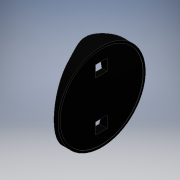
# Autodesk Inventor part: ET15
Saved by Autodesk Inventor 2016 (Build 200138000, 138)
## iProperties
Created: 2016-03-28
Part Number: ET15
Material: Genérico
Document SubType Name: Modeling
Designer: Usuario1
Density: 1 g/cm^3
Appearance: Valor por defecto
Author: Usuario1
Autodesk Inventor part; units mm, degrees
ref_plane "YZ Plane" through (0, 0, 0) normal (1, 0, 0) x (0, 1, 0)
ref_plane "XZ Plane" through (0, 0, 0) normal (0, 1, 0) x (-1, 0, 0)
ref_plane "XY Plane" through (0, 0, 0) normal (0, 0, 1) x (1, 0, 0)
sketch "Boceto4" plane through (0, 0, 0) normal (1, 0, 0) x (0, 1, 0)
  circle A0 centre (0, 0) radius 1.15
  circle A1 centre (0, 0) radius 1.0926
  constraints: 2 centre point
extrude "Extrusión3" add sketch "Boceto4" along normal blind 0.27 and the other way blind 0.155 contours A0 | A1
sketch "Boceto5" plane through (0, 0, 0) normal (0, 1, 0) x (-1, 0, 0)
  line L0 (-0.27, 1.15) -> (-0.27, -1.15) projected
  line L1 (0.155, -1.15) -> (0.155, 1.15) projected
  line L2 (0.155, -1.15) -> (0.155, 1.15) projected
  line L3 (0.155, -1.15) -> (-0.27, -1.15) projected
  line L4 (0.155, 1.15) -> (-0.27, 1.15) projected
  arc A0 (0.0009, 0.9764) -> (0.0009, -0.9764) centre (2.8, 0) ccw
  arc A1 (0.0009, -0.9764) -> (0.2382, -1.174) centre (0.2842, -0.8776) ccw
  arc A2 (0.2382, 1.174) -> (0.0009, 0.9764) centre (0.2842, 0.8776) ccw
  line L5 (0.2382, -1.174) -> (0.2382, 1.174)
  point P0 (0, 0)
  constraints: 6 point on circle, 3 centre point, 2 end point, 1 vertical, 1 other
extrude "Extrusión4" cut sketch "Boceto5" along normal mid plane 27 contours A2 L5 A1 L1 | L1 A1 A0 A2
sketch "Boceto6" plane through (0.27, 0, 0) normal (1, 0, 0) x (0, 0, -1)
  line L0 (0, 0) -> (0, 0.25)
  line L1 (0, 0.25) -> (0.25, 0.25)
  line L2 (0.25, 0.25) -> (0.25, -0.25)
  line L3 (0.25, -0.25) -> (-0.25, -0.25)
  line L4 (-0.25, -0.25) -> (-0.25, 0.25)
  line L5 (-0.25, 0.25) -> (0.25, 0.25)
  dimension "d10" = 0.25
  dimension "d11" = 0.25
  dimension "d12" = 0.5
  dimension "d13" = 0.5
  dimension "d14" = 0.5
  constraints: 12 end point, 4 perpendicular, 1 point on line, 1 vertical
  measures "d10" distance of L0.start L0.end
  measures "d11" distance of L0.end L1.end
  measures "d12" distance of L1.end L2.end
  measures "d13" distance of L2.end L3.end
  measures "d14" distance of L3.end L4.end
extrude "Extrusión5" add sketch "Boceto6" against normal blind 0.117
sketch "Boceto7" plane through (0.153, 0, 0) normal (-1, 0, 0) x (0, 0, 1)
  line L0 (-0.25, 0.25) -> (-0.25, -0.25) projected
  line L1 (-0.25, -0.25) -> (0.25, -0.25) projected
  line L2 (0.25, -0.25) -> (0.25, 0.25) projected
  line L3 (0.25, 0.25) -> (-0.25, 0.25) projected
  point P0 (0, 0)
extrude "Extrusión6" add sketch "Boceto7" along normal blind 0.5
sketch "Boceto8" plane through (0.27, 0, 0) normal (1, 0, 0) x (0, 0, -1)
  circle A0 centre (0, 0) radius 1.15
  circle A1 centre (0, 0) radius 1.0926
  constraints: 2 centre point
extrude "Extrusión7" cut sketch "Boceto8" against normal blind 0.01 contours A1
sketch "Boceto9" plane through (0.26, 0, 0) normal (1, 0, 0) x (0, 0, -1)
  line L0 (0.5, 0) -> (0.5, 0.15)
  line L1 (0.5, 0.15) -> (0.8, 0.15)
  line L2 (0.8, 0.15) -> (0.8, -0.15)
  line L3 (0.8, -0.15) -> (0.5, -0.15)
  line L4 (0.5, -0.15) -> (0.5, 0.15)
  line L5 (-0.5, 0) -> (-0.5, 0.15)
  line L6 (-0.5, 0.15) -> (-0.8, 0.15)
  line L7 (-0.8, 0.15) -> (-0.8, -0.15)
  line L8 (-0.8, -0.15) -> (-0.5, -0.15)
  line L9 (-0.5, -0.15) -> (-0.5, 0.15)
  point P0 (0, 0)
  dimension "d21" = 0.5
  dimension "d22" = 0.15
  dimension "d23" = 0.3
  dimension "d24" = 0.3
  dimension "d25" = 0.3
  constraints: 20 end point, 2 perpendicular, 2 point on line, 1 collinear
  measures "d21" distance of point (0, 0) L0.start
  measures "d22" distance of L0.start L0.end
  measures "d23" distance of L0.end L1.end
  measures "d24" distance of L1.end L2.end
  measures "d25" distance of L2.end L3.end
extrude "Extrusión8" cut sketch "Boceto9" against normal blind 0.3
